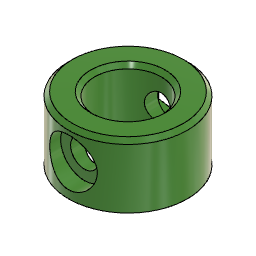
Picavet_Blocage_GLeguen_V0-0-2 (Autodesk Fusion 360 design; units mm, degrees)
Autodesk Fusion 360 part; units mm, degrees
sketch "Esquisse1" plane through (0, 0, 0) normal (0, 0, 1) x (1, 0, 0)
  circle A0 centre (0, 0) radius 4.2
  circle A1 centre (0, 0) radius 7.5
  dimension "d1" = 8.4
  dimension "d2" = 15
  constraint coincident A0.centre A1.centre
  measures "d1" diameter of A0
  measures "d2" diameter of A1
extrude "Extrusion1" add sketch "Esquisse1" along normal blind 8
hole "Perçage1" at (0, -7.5, 4) direction (0, 1, 0) diameter 3.5 depth 15 tip angle 180 counterbore diameter 6 counterbore depth 2
ref_plane "Plan de construction1" through (0, 7.5, 0) normal (0, 1, 0) x (0, 0, 1)
sketch "Esquisse2" plane through (0, 7.5, 0) normal (0, 1, 0) x (1, 0, 0)
  line L0 (-2.9935, -2.2568) -> (-3.0064, -5.7209)
  line L1 (-3.0064, -5.7209) -> (-0.0129, -7.4641)
  line L2 (-0.0129, -7.4641) -> (2.9935, -5.7432)
  line L3 (2.9935, -5.7432) -> (3.0064, -2.2791)
  line L4 (3.0064, -2.2791) -> (0.0129, -0.5359)
  line L5 (0.0129, -0.5359) -> (-2.9935, -2.2568)
  point P0 (0, -4)
  dimension "d12" = 3
  measures "d12" distance of P0 L5
extrude "Extrusion2" cut sketch "Esquisse2" against normal blind 2
chamfer "Chanfrein1" distance 0.5 angle 45 1 edges at (-3.9158, 1.5188, 8)
chamfer "Chanfrein2" distance 0.5 angle 45 1 edges at (-6.9925, -2.7121, 8)
